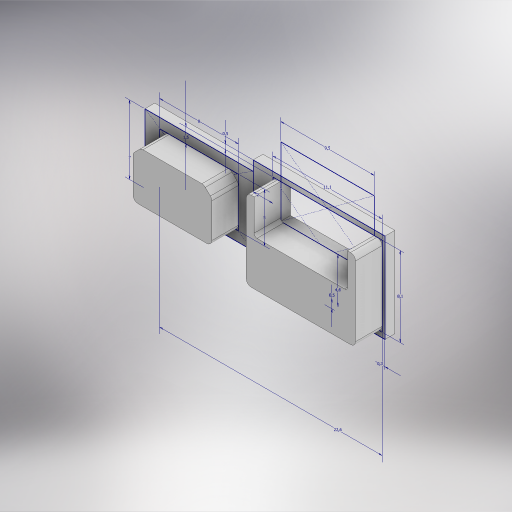
# Autodesk Inventor part: firewire-02
Saved by Autodesk Inventor 2024 (Build 280153000, 153)
## iProperties
Created: 2024-08-24
Part Number: firewire-02
Material: Generic
Document SubType Name: Modeling
Designer: User
Density: 1 g/cm^3
Appearance: Default
Author: User
Autodesk Inventor part; units mm, degrees
ref_plane "YZ Plane" through (0, 0, 0) normal (1, 0, 0) x (0, 1, 0)
ref_plane "XZ Plane" through (0, 0, 0) normal (0, 1, 0) x (-1, 0, 0)
ref_plane "XY Plane" through (0, 0, 0) normal (0, 0, 1) x (1, 0, 0)
sketch "Sketch1" plane through (0, 0, 0) normal (0, 0, 1) x (1, 0, 0)
  line L0 (-5.55, -4.05) -> (5.55, -4.05)
  line L1 (5.55, -4.05) -> (5.55, 4.05)
  line L2 (5.55, 4.05) -> (-5.55, 4.05)
  line L3 (-5.55, 4.05) -> (-5.55, -4.05)
  line L4 (-5.55, -4.05) -> (5.55, 4.05) construction
  line L5 (5.55, -4.05) -> (-5.55, 4.05) construction
  line L6 (-4.75, 0.55) -> (4.75, 0.55)
  line L7 (4.75, 0.55) -> (4.75, 7.55)
  line L8 (4.75, 7.55) -> (-4.75, 7.55)
  line L9 (-4.75, 7.55) -> (-4.75, 0.55)
  line L10 (-4.75, 0.55) -> (4.75, 7.55) construction
  line L11 (4.75, 0.55) -> (-4.75, 7.55) construction
  line L12 (5.85, -4.55) -> (-7.55, -4.55)
  line L13 (-7.55, -4.55) -> (-7.55, 4.55)
  line L14 (-7.55, 4.55) -> (5.85, 4.55)
  line L15 (5.85, 4.55) -> (5.85, -4.55)
  line L16 (-17.05, -2.45) -> (-9.05, -2.45)
  line L17 (-9.05, -2.45) -> (-9.05, 2.55)
  line L18 (-9.05, 2.55) -> (-17.05, 2.55)
  line L19 (-17.05, 2.55) -> (-17.05, -2.45)
  line L20 (-17.05, -2.45) -> (-9.05, 2.55) construction
  line L21 (-9.05, -2.45) -> (-17.05, 2.55) construction
  line L22 (-18.55, -3.45) -> (-7.55, -3.45)
  line L23 (-7.55, -3.45) -> (-7.55, 3.55)
  line L24 (-7.55, 3.55) -> (-18.55, 3.55)
  line L25 (-18.55, 3.55) -> (-18.55, -3.45)
  line L26 (-18.55, -3.45) -> (-7.55, 3.55) construction
  line L27 (-7.55, -3.45) -> (-18.55, 3.55) construction
  point P0 (0, 0)
  point P1 (0, 4.05)
  point P2 (4.75, 4.05)
  point P3 (-4.75, 4.05)
  point P4 (-13.05, 0.05)
  point P5 (-7.55, -3.45)
  dimension "d0" = 11.1
  dimension "d1" = 8.1
  dimension "d2" = 9.5
  dimension "d3" = 4.6
  dimension "d8" = 0.5
  dimension "d9" = 2
  dimension "d10" = 0.5
  dimension "d11" = 0.3
  dimension "d14" = 8
  dimension "d15" = 5
  dimension "d16" = 1.5
  dimension "d17" = 22.6
  dimension "d18" = 7
  constraints: 56 end point, 10 parallel, 9 midpoint, 5 horizontal, 5 perpendicular, 1 point on line
  measures "d0" distance of L2.end L1.end
  measures "d1" distance of L1.end L0.end
  measures "d2" distance of L8.end L7.end
  measures "d3" distance between parallel lines of L0 L6
  measures "d8" distance between parallel lines of L14 L2
  measures "d9" distance between parallel lines of L13 L3
  measures "d10" distance between parallel lines of L0 L12
  measures "d11" distance between parallel lines of L1 L15
  measures "d14" distance of L18.end L17.end
  measures "d15" distance of L17.end L16.end
  measures "d16" distance between parallel lines of L2 L18
  measures "d17" distance between parallel lines of L1 L19
  measures "d18" distance between parallel lines of L22 L24
extrude "Extrusion1" add sketch "Sketch1" along normal blind 2.7 contours L3 L2 L9 L6 L7 L1 L0
fillet "Fillet1" radius 0.5 4 edges at (5.55, 4.05, 1.35) (5.55, -4.05, 1.35) (-5.55, -4.05, 1.35) (-5.55, 4.05, 1.35)
fillet "Fillet2" radius 0.3 2 edges at (-4.75, 0.55, 1.35) (4.75, 0.55, 1.35)
extrude "Extrusion2" add sketch "Sketch1" against normal blind 1 contours L3 L2 L9 L6 L7 L1 L0 | L0 L1 L2 L7 L14 L15 L12 L13 L9 L3 | L9 L14 L7 L2
extrude "Extrusion3" add sketch "Sketch1" against normal up to surface (1 mm away) contours L13 L22 L25 L24 | L19 L18 L17 L16
extrude "Extrusion4" add sketch "Sketch1" along normal up to surface (2.7 mm away) contours L19 L18 L17 L16
chamfer "Chamfer1" distance 0.8 angle 45 2 edges at (-9.05, 2.55, 1.35) (-17.05, 2.55, 1.35)
fillet "Fillet3" radius 0.5 6 edges at (-9.85, 2.55, 1.35) (-9.05, 1.75, 1.35) (-9.05, -2.45, 1.35) (-16.25, 2.55, 1.35) (-17.05, 1.75, 1.35) (-17.05, -2.45, 1.35)
body "Solid1"
